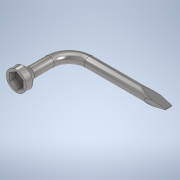
# Autodesk Inventor part: ключ
Saved by Autodesk Inventor 2020 (Build 240168000, 168)
## iProperties
Created: 2022-05-09
Part Number: ключ
Material: Сталь, гальванизированная
Document SubType Name: Modeling
Designer: User
Density: 7.85 g/cm^3
Appearance: Гальванизированная
Author: User
Autodesk Inventor part; units mm, degrees
ref_plane "YZ Plane" through (0, 0, 0) normal (1, 0, 0) x (0, 1, 0)
ref_plane "XZ Plane" through (0, 0, 0) normal (0, 1, 0) x (-1, 0, 0)
ref_plane "XY Plane" through (0, 0, 0) normal (0, 0, 1) x (1, 0, 0)
sketch "Эскиз1" plane through (0, 0, 0) normal (0, 1, 0) x (-1, 0, 0)
  line L0 (0, 0) -> (0, -30)
  line L1 (-30, -60) -> (-150, -60)
  arc A0 (-30, -60) -> (0, -30) centre (-30, -30) ccw
  point P0 (0, -60)
  dimension "d0" = 60
  dimension "d1" = 150
  dimension "d2" = 30
  constraints: 4 end point, 2 point on circle, 2 point on line, 2 tangent, 1 centre point, 1 perpendicular, 1 vertical
  measures "d0" distance of L0.start point (0, -60)
  measures "d1" distance of point (0, -60) L1.end
  measures "d2" radius of A0
sketch "Эскиз2" plane through (0, 0, 0) normal (0, 0, 1) x (1, 0, 0)
  circle A0 centre (0, 0) radius 7.5
  dimension "d3" = 15
  constraints: 1 centre point, 1 coincident
  measures "d3" diameter of A0
sweep "Сдвиг1" add profiles "Эскиз2" path "Эскиз1"
sketch "Эскиз3" plane through (0, 0, 0) normal (0, 1, 0) x (-1, 0, 0)
  line L0 (-120, -52.5) -> (-150, -55.1247)
  line L1 (-120, -67.5) -> (-150, -64.8753)
  line L2 (-150, -64.8753) -> (-150, -55.1247)
  line L3 (-150, -52.5) -> (-150, -67.5) projected
  line L4 (-120, -52.5) -> (-150.8821, -45.0422)
  line L5 (-150.8821, -45.0422) -> (-158.2895, -61.433)
  line L6 (-158.2895, -61.433) -> (-150, -78.5011)
  line L7 (-150, -78.5011) -> (-120, -67.5)
  point P0 (0, 0)
  constraints: 14 end point, 1 collinear, 1 point on line
extrude "Выдавливание1" cut sketch "Эскиз3" against normal mid plane 40
sketch "Эскиз4" plane through (0, 0, 0) normal (0, 0, 1) x (1, 0, 0)
  line L0 (30, 7.5) -> (150, 7.5) projected
  line L1 (110, 7.5) -> (150.3931, 7.5) construction
  line L2 (30, -7.5) -> (150, -7.5) projected
  line L3 (110, 7.5) -> (159.1062, 20.8998)
  line L4 (159.1062, 20.8998) -> (172.0854, -18.5057)
  line L5 (172.0854, -18.5057) -> (124.0272, -32.5373)
  line L6 (124.0272, -32.5373) -> (110, -7.5)
  line L7 (110, 7.5) -> (150, 0.4469)
  line L8 (150, -5.6992) -> (150, 5.6992) projected
  line L9 (110, 7.5) -> (150.6171, 7.5) construction
  line L10 (110, -7.5) -> (150, -0.4469)
  line L11 (150, 0.4469) -> (150, -0.4469)
  point P0 (0, 0)
  dimension "d13" = 10
  constraints: 18 end point, 2 horizontal, 2 point on line, 1 equal length, 1 vertical
  measures "d13" angle of L7 L9
extrude "Выдавливание2" cut sketch "Эскиз4" against normal blind 120
sketch "Эскиз5" plane through (0, 0, 0) normal (0, 1, 0) x (-1, 0, 0)
  line L0 (0, 0) -> (0, 20)
  line L1 (0, 20) -> (15, 20)
  line L2 (15, 20) -> (15, 10)
  line L3 (7.5, 0) -> (-7.5, 0) projected
  line L4 (7.5, 0) -> (15, 10)
  dimension "d14" = 20
  dimension "d15" = 15
  dimension "d16" = 10
  constraints: 8 end point, 1 horizontal, 1 perpendicular, 1 vertical
  measures "d14" distance of L0.start L0.end
  measures "d15" distance of L0.end L1.end
  measures "d16" distance of L1.end L2.end
revolve "Вращение1" add sketch "Эскиз5" angle 360 about axis through (0, 0, 0) along (0, 0, 1)
sketch "Эскиз10" plane through (0, 0, 20) normal (0, 0, 1) x (1, 0, 0)
  line L0 (0, 12.1042) -> (10.4826, 6.0521)
  line L1 (10.4826, 6.0521) -> (10.4826, -6.0521)
  line L2 (10.4826, -6.0521) -> (0, -12.1042)
  line L3 (0, -12.1042) -> (-10.4826, -6.0521)
  line L4 (-10.4826, -6.0521) -> (-10.4826, 6.0521)
  line L5 (-10.4826, 6.0521) -> (0, 12.1042)
  point P0 (0, 0)
  point P1 (0, 0)
  constraints: 12 end point, 1 coincident, 13 other
extrude "Выдавливание3" cut sketch "Эскиз10" against normal blind 10
